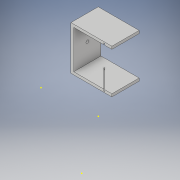
# Autodesk Inventor part: Spiegelhalter Objekthalter 1
Saved by Autodesk Inventor 2017 (Build 210142000, 142)
## iProperties
Part Number: Spiegelhalter Objekthalter 1
Material: Generisch
Document SubType Name: Modeling
Designer: pgmadmin
Density: 1 g/cm^3
Appearance: Vorgabe
Author: pgmadmin
Autodesk Inventor part; units mm, degrees
ref_plane "YZ Plane" through (0, 0, 0) normal (1, 0, 0) x (0, 1, 0)
ref_plane "XZ Plane" through (0, 0, 0) normal (0, 1, 0) x (-1, 0, 0)
ref_plane "XY Plane" through (0, 0, 0) normal (0, 0, 1) x (1, 0, 0)
sketch "Skizze1" plane through (0, 0, 0) normal (1, 0, 0) x (0, 1, 0)
  line L0 (105.1634, 173.9786) -> (55.1634, 173.9786)
  line L1 (55.1634, 173.9786) -> (55.1634, 93.4786)
  line L2 (55.1634, 93.4786) -> (105.1634, 93.4786)
  line L3 (105.1634, 93.4786) -> (105.1634, 173.9786)
  point P0 (0, 0)
  dimension "d0" = 80.5
  dimension "d1" = 50
  constraints: 8 end point, 2 parallel, 1 horizontal, 1 perpendicular
  measures "d0" distance of L2.end L0.start
  measures "d1" distance of L1.end L2.end
extrude "Extrusion1" add sketch "Skizze1" along normal blind 5
sketch "Skizze2" plane through (5, 0, 0) normal (1, 0, 0) x (0, 0, -1)
  line L0 (-173.9786, 105.1639) -> (-168.9786, 105.1634)
  line L1 (-93.4786, 105.1634) -> (-173.9786, 105.1634) projected
  line L2 (-173.9786, 55.1634) -> (-93.4786, 55.1634) projected
  line L3 (-168.9786, 55.1634) -> (-173.9786, 55.1634)
  line L4 (-173.9786, 55.1634) -> (-173.9786, 105.1639)
  line L5 (-168.9786, 105.1634) -> (-168.9786, 55.1634)
  line L6 (-93.4786, 105.1634) -> (-98.4786, 105.1634)
  line L7 (-98.4786, 55.1634) -> (-93.4786, 55.1634)
  line L8 (-93.4786, 55.1634) -> (-93.4786, 105.1634) projected
  line L9 (-93.4786, 105.1634) -> (-98.4786, 105.1634)
  line L10 (-98.4786, 55.1634) -> (-98.4786, 105.1634)
  line L11 (-98.4786, 105.1634) -> (-93.4786, 105.1634)
  line L12 (-93.4786, 55.1634) -> (-98.4786, 55.1634)
  line L13 (-98.4786, 105.1634) -> (-93.4786, 105.1634)
  line L14 (-93.4786, 55.1634) -> (-98.4786, 55.1634)
  line L15 (-98.4786, 105.1634) -> (-93.4786, 105.1634)
  point P0 (0, 0)
  dimension "d4" = 5
  dimension "d5" = 5
  constraints: 26 end point, 5 parallel, 4 perpendicular, 4 point on line, 1 collinear, 1 horizontal
  measures "d4" distance of L0.start L0.end
  measures "d5" distance between parallel lines of L8 L10
extrude "Extrusion2" add sketch "Skizze2" along normal blind 70 contours L1 L8 L2 L10
sketch "Skizze3" plane through (5, 55.1634, 98.4786) normal (0, 0, 1) x (1, 0, 0)
  line L0 (22.2218, 34.8995) -> (57.5772, -0.4558)
  line L1 (57.5772, -0.4558) -> (56.5165, -1.5165)
  line L2 (56.5165, -1.5165) -> (21.1612, 33.8388)
  line L3 (21.1612, 33.8388) -> (22.2218, 34.8995)
  line L4 (-5, 50) -> (-5, 0) projected
  line L5 (21.1612, 33.8388) -> (38.8388, 16.1612)
  line L6 (0, 50) -> (70, 50) projected
  line L7 (57.5772, -0.4558) -> (56.5165, -1.5165)
  line L8 (56.5165, -1.5165) -> (57.5772, -0.4558)
  line L9 (51.6127, 5.5086) -> (50.5521, 4.4479)
  line L10 (50.5521, 4.4479) -> (56.5165, -1.5165)
  line L11 (57.5772, -0.4558) -> (51.6127, 5.5086)
  point P0 (-5, -55.1634)
  dimension "d8" = 1.5
  dimension "d9" = 50
  dimension "d10" = 45
  dimension "d35" = 16.1612
  dimension "d36" = 26.1612
  constraints: 20 end point, 5 perpendicular, 2 equal length, 2 point on line, 1 midpoint
  measures "d8" distance of L0.end L1.end
  measures "d9" distance of L0.start L0.end
  measures "d10" angle of L4 L2
  measures "d35" distance from line of L6 L2.end
  measures "d36" distance from line of L4 L2.end
sketch "Skizze4" plane through (0, 105.1634, 173.9786) normal (0, 1, 0) x (1, 0, 0)
  point P0 (0, 173.9786)
extrude "Extrusion3" cut sketch "Skizze3" against normal blind 3
sketch "Skizze5" plane through (5, 0, 0) normal (1, 0, 0) x (0, 0, -1)
  line L0 (-173.9786, 105.1634) -> (-173.9786, 55.1634) projected
  line L1 (-173.9786, 55.1634) -> (-168.9786, 55.1634)
  line L2 (-173.9786, 55.1634) -> (-98.4786, 55.1634) projected
  line L3 (-98.4786, 105.1634) -> (-173.9786, 105.1634) projected
  line L4 (-168.9786, 105.1634) -> (-173.9786, 105.1634)
  line L5 (-173.9786, 105.1634) -> (-173.9786, 55.1634)
  line L6 (-168.9786, 55.1634) -> (-168.9786, 105.1634)
  point P0 (0, 0)
  dimension "d15" = 5
  constraints: 8 end point, 2 point on line, 1 horizontal, 1 parallel, 1 perpendicular
  measures "d15" distance of L0.end L1.end
extrude "Extrusion4" add sketch "Skizze5" along normal blind 70
sketch "Skizze6" plane through (5, 55.1634, 168.9786) normal (0, 0, -1) x (-1, 0, 0)
  line L0 (-57.5772, -0.4558) -> (-56.5165, -1.5165)
  line L1 (-56.5165, -1.5165) -> (-21.1612, 33.8388)
  line L2 (-21.1612, 33.8388) -> (-22.2218, 34.8995)
  line L3 (-22.2218, 34.8995) -> (-57.5772, -0.4558)
  line L4 (0, 50) -> (0, 0) projected
  line L5 (-21.1612, 33.8388) -> (-38.8388, 16.1612)
  line L6 (0, 0) -> (-70, 0) projected
  line L7 (-56.5165, -1.5165) -> (-57.5772, -0.4558)
  line L8 (-53.774, 3.3474) -> (-52.7133, 2.2867)
  line L9 (-52.7133, 2.2867) -> (-56.5165, -1.5165)
  line L10 (-57.5772, -0.4558) -> (-53.774, 3.3474)
  line L11 (0, 50) -> (-70, 50) projected
  point P0 (5, -55.1634)
  dimension "d18" = 1.5
  dimension "d19" = 50
  dimension "d20" = 45
  dimension "d22" = 1.5
  dimension "d37" = 21.1612
  dimension "d38" = 16.1612
  constraints: 18 end point, 3 perpendicular, 2 parallel, 1 midpoint
  measures "d18" distance of L0.start L0.end
  measures "d19" distance of L0.end L1.end
  measures "d20" angle of L4 L1
  measures "d22" distance of L1.end L2.end
  measures "d37" distance from line of L4 L1.end
  measures "d38" distance from line of L11 L1.end
extrude "Extrusion5" cut sketch "Skizze6" against normal blind 3
sketch "Skizze7" plane through (75, 0, 0) normal (1, 0, 0) x (0, 0, -1)
  point P0 (0, 0)
sketch "Skizze8" plane through (75, 0, 0) normal (1, 0, 0) x (0, 0, -1)
  point P0 (0, 0)
sketch "Skizze9" plane through (0, 0, 0) normal (-1, 0, 0) x (0, 0, 1)
  line L0 (93.4786, 55.1634) -> (93.4786, 105.1634) projected
  line L1 (93.4786, 105.1634) -> (173.9786, 105.1634) projected
  point P0 (0, 0)
  point P1 (133.7286, 80.1634)
  dimension "d26" = 40.25
  dimension "d27" = 25
  measures "d26" distance from line of L0 point (133.729, 80.163)
  measures "d27" distance from line of L1 point (133.729, 80.163)
hole "Bohrung1" at (0, 80.1634, 133.7286) direction (1, 0, 0) diameter 5 end through all
sketch "Skizze10" plane through (5, 55.1634, 98.4786) normal (0, 0, 1) x (1, 0, 0)
  point P0 (-5, -55.1634)
